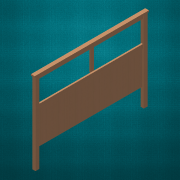
# Autodesk Inventor part: Footer
Saved by Autodesk Inventor 2017 (Build 210142000, 142)
## iProperties
Created: 2017-06-03
Part Number: Footer
Material: Wood (Cherry)
Document SubType Name: Modeling
Designer: Michael
Density: 0.63 g/cm^3
Appearance: Cherry - Natural Low Gloss
Author: Michael
Autodesk Inventor part; units mm, degrees
ref_plane "YZ Plane" through (0, 0, 0) normal (1, 0, 0) x (0, 1, 0)
ref_plane "XZ Plane" through (0, 0, 0) normal (0, 1, 0) x (-1, 0, 0)
ref_plane "XY Plane" through (0, 0, 0) normal (0, 0, 1) x (1, 0, 0)
sketch "Sketch1" plane through (0, 0, 0) normal (0, 1, 0) x (-1, 0, 0)
  line L0 (-23.8125, 811.2125) -> (23.8125, 811.2125)
  line L1 (23.8125, 811.2125) -> (23.8125, 754.0625)
  line L2 (23.8125, 754.0625) -> (-23.8125, 754.0625)
  line L3 (-23.8125, 754.0625) -> (-23.8125, 811.2125)
  line L4 (-23.8125, 811.2125) -> (23.8125, 754.0625) construction
  line L5 (23.8125, 811.2125) -> (-23.8125, 754.0625) construction
  line L6 (-23.8125, -754.0625) -> (23.8125, -754.0625)
  line L7 (23.8125, -754.0625) -> (23.8125, -811.2125)
  line L8 (23.8125, -811.2125) -> (-23.8125, -811.2125)
  line L9 (-23.8125, -811.2125) -> (-23.8125, -754.0625)
  line L10 (-23.8125, -754.0625) -> (23.8125, -811.2125) construction
  line L11 (23.8125, -754.0625) -> (-23.8125, -811.2125) construction
  line L12 (0, 754.0625) -> (0, 0) construction
  line L13 (0, 0) -> (0, -754.0625) construction
  point P0 (0, 782.6375)
  point P1 (0, -782.6375)
  point P2 (0, 782.6375)
  point P3 (0, -782.6375)
  dimension "d0" = 47.625
  dimension "d1" = 57.15
  dimension "d2" = 1622.425
  constraints: 28 end point, 8 midpoint, 4 parallel, 3 equal length, 2 horizontal, 2 perpendicular, 2 vertical alignment, 1 point on line, 1 vertical
  measures "d0" distance of L0.start L0.end
  measures "d1" distance of L0.end L1.end
  measures "d2" distance between parallel lines of L8 L0
extrude "Extrusion1" add sketch "Sketch1" along normal blind 1174.75
sketch "Sketch2" plane through (0, 0, 0) normal (0, 0, 1) x (1, 0, 0)
  line L0 (-26.9875, 1196.975) -> (26.9875, 1196.975)
  line L1 (26.9875, 1196.975) -> (26.9875, 1174.75)
  line L2 (26.9875, 1174.75) -> (-26.9875, 1174.75)
  line L3 (-26.9875, 1174.75) -> (-26.9875, 1196.975)
  line L4 (-26.9875, 1196.975) -> (26.9875, 1174.75) construction
  line L5 (26.9875, 1196.975) -> (-26.9875, 1174.75) construction
  line L6 (23.8125, 0) -> (-23.8125, 0) projected
  point P0 (0, 0)
  point P1 (0, 1185.8625)
  point P2 (-23.8125, 1174.75)
  point P3 (0, 1185.8625)
  point P4 (0, 0)
  dimension "d5" = 53.975
  dimension "d6" = 22.225
  constraints: 12 end point, 4 midpoint, 2 parallel, 1 horizontal, 1 perpendicular, 1 point on line, 1 vertical alignment
  measures "d5" distance of L0.start L0.end
  measures "d6" distance of L0.end L1.end
extrude "Extrusion2" add sketch "Sketch2" along normal mid plane 1651
sketch "Sketch3" plane through (0, 0, 0) normal (0, 0, 1) x (1, 0, 0)
  line L0 (23.8125, 1174.75) -> (-23.8125, 1174.75) projected
  line L1 (11.1125, 1117.6) -> (-11.1125, 1117.6)
  line L2 (-11.1125, 1117.6) -> (-11.1125, 1174.75)
  line L3 (-11.1125, 1174.75) -> (11.1125, 1174.75)
  line L4 (11.1125, 1174.75) -> (11.1125, 1117.6)
  line L5 (11.1125, 1117.6) -> (-11.1125, 1174.75) construction
  line L6 (-11.1125, 1117.6) -> (11.1125, 1174.75) construction
  line L7 (11.1125, 746.125) -> (-11.1125, 746.125)
  line L8 (-11.1125, 746.125) -> (-11.1125, 803.275)
  line L9 (-11.1125, 803.275) -> (11.1125, 803.275)
  line L10 (11.1125, 803.275) -> (11.1125, 746.125)
  line L11 (11.1125, 746.125) -> (-11.1125, 803.275) construction
  line L12 (-11.1125, 746.125) -> (11.1125, 803.275) construction
  line L13 (-3.175, 203.2) -> (3.175, 203.2)
  line L14 (3.175, 203.2) -> (3.175, 746.125)
  line L15 (3.175, 746.125) -> (-3.175, 746.125)
  line L16 (-3.175, 746.125) -> (-3.175, 203.2)
  line L17 (-3.175, 203.2) -> (3.175, 746.125) construction
  line L18 (3.175, 203.2) -> (-3.175, 746.125) construction
  line L19 (23.8125, 0) -> (-23.8125, 0) projected
  point P0 (0, 0)
  point P1 (0, 1146.175)
  point P2 (0, 1146.175)
  point P3 (0, 1174.75)
  point P4 (0, 774.7)
  point P5 (0, 774.7)
  point P6 (0, 474.6625)
  point P7 (0, 774.7)
  point P8 (0, 474.6625)
  dimension "d9" = 57.15
  dimension "d10" = 22.225
  dimension "d22" = 6.35
  dimension "d23" = 203.2
  dimension "d30" = 314.325
  constraints: 36 end point, 11 midpoint, 6 parallel, 3 horizontal, 3 perpendicular, 3 vertical alignment, 2 equal length, 2 point on line
  measures "d9" distance of L1.end L2.end
  measures "d10" distance between parallel lines of L2 L4
  measures "d22" distance between parallel lines of L14 L16
  measures "d23" distance between parallel lines of L19 L13
  measures "d30" distance between parallel lines of L1 L9
extrude "Extrusion3" add sketch "Sketch3" against normal up to surface (1508.125 mm away) from surface at 754.0625 contours L4 L1 L2 L0 | L7 L8 L9 L10
sketch "Sketch4" plane through (-11.1125, 803.275, 754.0625) normal (0, 1, 0) x (1, 0, 0)
  line L0 (17.4625, 661.9875) -> (4.7625, 661.9875)
  line L1 (4.7625, 661.9875) -> (4.7625, 719.1375)
  line L2 (4.7625, 719.1375) -> (17.4625, 719.1375)
  line L3 (17.4625, 719.1375) -> (17.4625, 661.9875)
  line L4 (17.4625, 661.9875) -> (4.7625, 719.1375) construction
  line L5 (4.7625, 661.9875) -> (17.4625, 719.1375) construction
  line L6 (14.2875, 661.9875) -> (7.9375, 661.9875)
  line L7 (14.2875, 719.1375) -> (7.9375, 719.1375)
  line L8 (0, 0) -> (0, 1508.125) projected
  line L9 (0, 0) -> (0, 1508.125) projected
  line L10 (0, 1508.125) -> (22.225, 1508.125) projected
  point P0 (11.1125, 690.5625)
  point P1 (11.1125, 690.5625)
  point P2 (11.1125, 690.5625)
  point P3 (0, 754.0625)
  point P4 (11.1125, 1508.125)
  dimension "d15" = 12.7
  dimension "d16" = 57.15
  dimension "d34" = 63.5
  constraints: 16 end point, 6 midpoint, 3 parallel, 2 point on line, 1 horizontal, 1 perpendicular, 1 vertical alignment
  measures "d15" distance of L1.end L2.end
  measures "d16" distance of L0.end L1.end
  measures "d34" vertical distance of point (11.113, 690.563) point (0, 754.063)
extrude "Extrusion4" add sketch "Sketch4" along normal up to next separate body
chamfer "Chamfer1" distance 1.5875 angle 45 12 edges at (11.1125, 1117.6, 0) (11.1125, 803.275, 0) (-11.1125, 1117.6, 0) (-11.1125, 803.275, 0) (6.35, 960.4375, 92.075) (6.35, 1117.6, 63.5) (6.35, 960.4375, 34.925) (6.35, 803.275, 63.5) (-6.35, 960.4375, 34.925) (-6.35, 1117.6, 63.5) (-6.35, 960.4375, 92.075) (-6.35, 803.275, 63.5)
pattern_linear "Rectangular Pattern1" count 4 spacing 127 along (0, 0, 1) count 5 spacing 127 along (0, 0, -1) bodies 2
sketch "Sketch5" plane through (11.1125, 746.125, -754.0625) normal (0, -1, 0) x (1, 0, 0)
  line L0 (-14.2875, 1508.125) -> (-7.9375, 1508.125)
  line L1 (-7.9375, 1508.125) -> (-7.9375, 0)
  line L2 (-7.9375, 0) -> (-14.2875, 0)
  line L3 (-14.2875, 0) -> (-14.2875, 1508.125)
  line L4 (-14.2875, 1508.125) -> (-7.9375, 0) construction
  line L5 (-7.9375, 1508.125) -> (-14.2875, 0) construction
  line L6 (12.7, 0) -> (-34.925, 0) projected
  point P0 (-11.1125, 754.0625)
  dimension "d27" = 6.35
  constraints: 12 end point, 2 midpoint, 2 parallel, 1 horizontal, 1 perpendicular, 1 point on line
  measures "d27" distance between parallel lines of L3 L1
extrude "Extrusion5" add sketch "Sketch5" along normal blind 482.6 bodies 1
body "Solid1"
body "Solid2"
